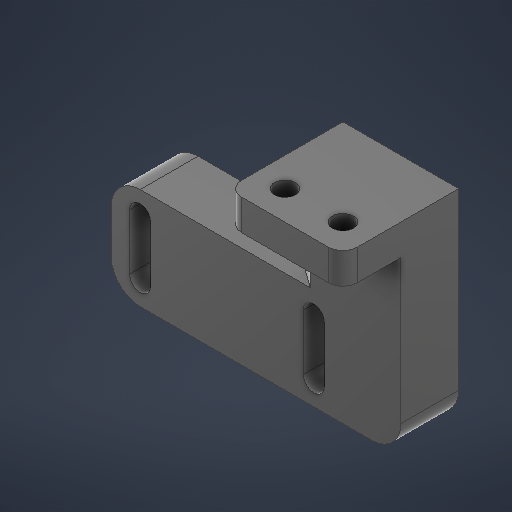
# Autodesk Inventor part: Optical Mount
Saved by Autodesk Inventor 2025 (Build 290162000, 162)
## iProperties
Created: 2024-12-22
Part Number: Optical Mount
Material: Generic
Document SubType Name: Modeling
Designer: Juan
Density: 1 g/cm^3
Appearance: Default
Author: Juan
Autodesk Inventor part; units mm, degrees
ref_plane "YZ Plane" through (0, 0, 0) normal (1, 0, 0) x (0, 1, 0)
ref_plane "XZ Plane" through (0, 0, 0) normal (0, 1, 0) x (-1, 0, 0)
ref_plane "XY Plane" through (0, 0, 0) normal (0, 0, 1) x (1, 0, 0)
sketch "Sketch1" plane through (0, 0, 0) normal (0, 0, 1) x (1, 0, 0)
  line L0 (-19.1352, -8.5102) -> (-19.1352, 8.3898) construction
  line L1 (-16.8111, -6.1861) -> (-16.8111, 6.0657)
  line L2 (-21.4593, 6.0657) -> (-21.4593, -6.1861)
  arc A0 (-21.4593, -6.1861) -> (-16.8111, -6.1861) centre (-19.1352, -6.1861) ccw
  arc A1 (-16.8111, 6.0657) -> (-21.4593, 6.0657) centre (-19.1352, 6.0657) ccw
  line L3 (18.9648, -8.5102) -> (18.9648, 8.3898) construction
  line L4 (21.2889, -6.1861) -> (21.2889, 6.0657)
  line L5 (16.6407, 6.0657) -> (16.6407, -6.1861)
  arc A2 (16.6407, -6.1861) -> (21.2889, -6.1861) centre (18.9648, -6.1861) ccw
  arc A3 (21.2889, 6.0657) -> (16.6407, 6.0657) centre (18.9648, 6.0657) ccw
  line L6 (-19.1352, 8.3898) -> (18.9648, 8.3898)
  line L7 (18.9648, -8.5102) -> (-19.1352, -8.5102)
  line L8 (25.3148, 11.0523) -> (-25.4852, 11.0523)
  line L9 (-25.4852, 11.0523) -> (-25.4852, -11.1727)
  line L10 (-25.4852, -11.1727) -> (25.3148, -11.1727)
  line L11 (25.3148, -11.1727) -> (25.3148, 11.0523)
  line L12 (25.3148, 11.0523) -> (-25.4852, -11.1727) construction
  line L13 (-25.4852, 11.0523) -> (25.3148, -11.1727) construction
  point P0 (0, 0)
  point P1 (-0.0852, -0.0602)
  point P2 (-19.1352, -0.0602)
  point P3 (18.9648, -0.0602)
  dimension "d0" = 4.6482
  dimension "d1" = 4.6482
  dimension "d2" = 50.8
  dimension "d3" = 22.225
  constraints: 32 end point, 12 point on circle, 10 tangent, 5 parallel, 4 centre point, 4 midpoint, 4 point on line, 2 perpendicular, 1 horizontal, 1 other
  measures "d0" diameter of A1
  measures "d1" diameter of A3
  measures "d2" distance of L10.end L9.end
  measures "d3" distance of L9.end L8.end
extrude "Extrusion1" add sketch "Sketch1" along normal blind 12.7 contours L1 A1 L6 A3 L5 A2 L7 A0 | L11 L10 L9 L8
sketch "Sketch2" plane through (-25.4852, 11.0523, 0) normal (0, 1, 0) x (1, 0, 0)
  line L0 (0, 0) -> (50.8, 0) projected
  line L1 (0, 0) -> (12.7, 0)
  line L2 (12.7, 0) -> (12.7, -12.7)
  line L3 (12.7, -12.7) -> (0, -12.7)
  line L4 (0, -12.7) -> (0, 0)
  line L5 (50.8073, 0) -> (38.1073, 0)
  line L6 (38.1073, 0) -> (38.1073, -12.7)
  line L7 (38.1073, -12.7) -> (50.8073, -12.7)
  line L8 (50.8, 0) -> (50.8, -12.7) projected
  line L9 (50.8, 0) -> (50.8, -12.7) projected
  line L10 (50.8, -12.7) -> (50.8, 0)
  line L11 (50.8, 0) -> (38.1073, 0)
  point P0 (25.4852, 0)
  dimension "d7" = 12.7
  dimension "d8" = 12.7
  dimension "d9" = 12.7
  dimension "d10" = 12.7
  constraints: 18 end point, 3 parallel, 3 perpendicular, 3 point on line, 1 collinear
  measures "d7" distance of L2.end L3.end
  measures "d8" distance of L6.end L7.end
  measures "d9" distance of L7.end L5.start
  measures "d10" distance of L3.end L0.start
extrude "Extrusion2" add sketch "Sketch2" along normal blind 22.3933
chamfer "Chamfer1" distance 3.9688 distance2 5.5563 1 edges at (12.6221, 22.2489, 12.7) measured on face at (12.6221, 22.2489, 12.2)
chamfer "Chamfer2" distance 4.7625 distance2 7.9375 1 edges at (-12.7852, 22.2489, 0) measured on face at (-12.7852, 22.2489, 0.5)
sketch "Sketch3" plane through (-25.4852, 33.4456, 0) normal (0, 1, 0) x (1, 0, 0)
  line L0 (0, 0) -> (6.319, 0)
  line L1 (38.1073, 0) -> (4.7625, 0) projected
  line L2 (6.319, -0.6519) -> (0, -0.6519)
  line L3 (0, 0) -> (0, -12.7) projected
  line L4 (0, 0) -> (0, -0.6519)
  line L5 (6.319, 0) -> (6.319, -0.6519)
  point P0 (25.4852, 0)
  constraints: 8 end point, 2 point on line, 1 collinear, 1 parallel, 1 perpendicular
extrude "Extrusion3" cut sketch "Sketch3" against normal up to surface (22.3933 mm away)
fillet "Fillet2" radius 3.175 2 edges at (-19.6363, 22.2489, 0.6519) (-25.4852, 22.2489, 0.6519)
sketch "Sketch4" plane through (0, 0, 12.7) normal (0, 0, 1) x (1, 0, 0)
  line L0 (-12.7852, 11.0523) -> (-18.8822, 11.0523) projected
  line L1 (-12.7852, 11.0523) -> (-12.7852, 26.6987)
  line L2 (-12.7852, 33.4456) -> (-12.7852, 11.0523) projected
  line L3 (-12.7852, 11.0523) -> (25.3148, 11.0523)
  line L4 (25.3148, -11.1727) -> (25.3148, 33.4456) projected
  line L5 (25.3148, 11.0523) -> (25.3148, 26.6987)
  line L6 (12.6221, 33.4456) -> (12.6221, 11.0523) projected
  line L7 (-25.4852, -11.1727) -> (-25.4852, 33.4456) projected
  line L8 (25.3148, 26.6987) -> (12.6221, 26.6987)
  line L9 (12.6221, 26.6987) -> (12.6221, 36.2237)
  line L10 (25.3148, 36.2237) -> (25.3148, 26.6987)
  line L11 (-12.7852, 26.6987) -> (-25.4852, 26.6987)
  line L12 (-25.4852, 26.6987) -> (-25.4852, 36.2237)
  line L13 (-12.7852, 36.2237) -> (-12.7852, 26.6987)
  line L14 (18.1783, 33.4456) -> (12.6221, 33.4456) projected
  line L15 (25.3148, 33.4456) -> (12.6221, 33.4456)
  line L16 (-12.7852, 36.2237) -> (-12.7852, 33.4456)
  line L17 (-25.4852, 33.4456) -> (-12.7852, 33.4456) projected
  line L18 (-12.7852, 33.4456) -> (-25.4852, 33.4456)
  line L19 (-25.4852, 33.4456) -> (-25.4852, 36.2237)
  line L20 (12.6221, 33.4456) -> (12.6221, 26.6987)
  line L21 (25.3148, 26.6987) -> (25.3148, 33.4456)
  line L22 (-12.7852, 26.6987) -> (-12.7852, 33.4456)
  line L23 (-25.4852, 26.6987) -> (-25.4852, 33.4456)
  point P0 (0, 0)
  dimension "d22" = 15.6464
  constraints: 34 end point, 6 perpendicular, 6 point on line, 4 parallel, 3 collinear, 1 horizontal
  measures "d22" distance of L0.start L1.end
extrude "Extrusion4" add sketch "Sketch4" along normal blind 12.7 contours L2 L11 L7 L17 | L6 L14 L15 L4 L8
extrude "Extrusion5" add sketch "Sketch4" against normal blind 4.2333 contours L6 L14 L15 L4 L8
sketch "Sketch5" plane through (-25.4852, 33.4456, 0) normal (0, 1, 0) x (1, 0, 0)
  line L0 (50.8, -25.4) -> (38.1073, -25.4) projected
  line L1 (12.7, -25.4) -> (0, -25.4) projected
  line L2 (44.4537, -25.4) -> (44.4537, -19.05)
  line L3 (6.35, -25.4) -> (6.35, -19.05)
  circle A0 centre (6.35, -19.05) radius 2.3241
  circle A1 centre (44.4537, -19.05) radius 2.3241
  point P0 (25.4852, 0)
  dimension "d27" = 6.35
  dimension "d28" = 6.35
  dimension "d29" = 4.6482
  dimension "d30" = 4.6482
  constraints: 4 end point, 2 centre point, 2 coincident, 2 midpoint, 2 vertical
  measures "d27" distance of L2.start L2.end
  measures "d28" distance of L3.start L3.end
  measures "d29" diameter of A0
  measures "d30" diameter of A1
extrude "Extrusion6" cut sketch "Sketch5" against normal through all
sketch "Sketch6" plane through (-12.7852, 11.0523, 12.7) normal (1, 0, 0) x (0, 0, -1)
  line L0 (-12.7, 15.6464) -> (-12.7, 22.3933) projected
  line L1 (0, 15.6464) -> (-12.7, 15.6464) projected
  line L2 (-12.7, 15.6464) -> (-12.7, 22.3933)
  line L3 (-12.7, 22.3933) -> (0, 22.3933)
  line L4 (0, 22.3933) -> (0, 15.6464)
  line L5 (0, 15.6464) -> (-12.7, 15.6464)
  point P0 (12.7, -11.0523)
  constraints: 8 end point, 3 equal length, 1 perpendicular
extrude "Extrusion7" [suppressed]
sketch "Sketch7" plane through (18.1783, 26.6987, 12.7) normal (0, -1, 0) x (1, 0, 0)
  circle A0 centre (-37.3136, 6.35) radius 2.3241 projected
  circle A1 centre (0.7901, 6.35) radius 2.3241 projected
  line L0 (-37.3136, 6.35) -> (-24.6136, 6.35)
  line L1 (-24.6136, 6.35) -> (-11.9136, 6.35)
  line L2 (-26.798, 4.1656) -> (-22.4292, 4.1656)
  line L3 (-22.4292, 4.1656) -> (-22.4292, 8.5344)
  line L4 (-22.4292, 8.5344) -> (-26.798, 8.5344)
  line L5 (-26.798, 8.5344) -> (-26.798, 4.1656)
  line L6 (-26.798, 4.1656) -> (-22.4292, 8.5344) construction
  line L7 (-22.4292, 4.1656) -> (-26.798, 8.5344) construction
  line L8 (-9.7292, 8.5344) -> (-14.098, 8.5344)
  line L9 (-9.7292, 4.1656) -> (-9.7292, 8.5344)
  line L10 (-14.098, 4.1656) -> (-9.7292, 4.1656)
  line L11 (-14.098, 8.5344) -> (-14.098, 4.1656)
  point P0 (-18.1783, -12.7)
  dimension "d35" = 12.7
  dimension "d36" = 12.7
  dimension "d37" = 4.3688
  dimension "d38" = 4.3688
  dimension "d41" = 12.7
  constraints: 24 end point, 3 horizontal, 2 midpoint, 2 parallel, 1 perpendicular, 1 point on line, 8 other
  measures "d35" distance of L0.start L0.end
  measures "d36" distance of L0.end L1.end
  measures "d37" distance of L4.end L3.end
  measures "d38" distance of L3.end L2.end
  measures "d41" distance of L3.end L8.start
extrude "Extrusion8" [suppressed]
fillet "Fillet3" [suppressed]
sketch "Sketch8" plane through (-25.4852, 11.0523, 0) normal (0, 1, 0) x (1, 0, 0)
  line L0 (38.1073, 0) -> (0, 0) projected
  line L1 (0, 0) -> (14.6548, 0)
  line L2 (14.6548, 0) -> (14.6548, -26.951)
  line L3 (14.6548, -26.951) -> (0, -26.951)
  line L4 (0, -26.951) -> (0, 0)
  point P0 (25.4852, 0)
  point P1 (14.6548, 0)
  constraints: 8 end point, 2 parallel, 1 horizontal, 1 perpendicular
extrude "Extrusion9" cut sketch "Sketch8" along normal blind 25.4
sketch "Sketch9" plane through (25.3148, -11.1727, 12.7) normal (1, 0, 0) x (0, 0, -1)
  line L0 (0, 0) -> (0, 37.8714) projected
  line L1 (12.7, 0) -> (0, 0) projected
  line L2 (12.7, 0) -> (12.7, 44.6183) projected
  line L3 (12.7, 44.6183) -> (-12.7, 44.6183) projected
  line L4 (-12.7, 37.8714) -> (-12.7, 44.6183) projected
  line L5 (0, 37.8714) -> (-12.7, 37.8714) projected
  point P0 (12.7, 11.1727)
extrude "Extrusion10" add sketch "Sketch9" along normal blind 12.7
sketch "Sketch10" plane through (-25.4852, 33.4456, 0) normal (0, 1, 0) x (1, 0, 0)
  circle A0 centre (44.4537, -19.05) radius 2.3241 projected
  line L0 (44.4537, -19.05) -> (57.1537, -19.05)
  circle A1 centre (57.1537, -19.05) radius 2.3241
  point P0 (25.4852, 0)
  dimension "d58" = 12.7
  dimension "d59" = 4.6482
  constraints: 2 end point, 1 centre point, 1 coincident, 1 horizontal
  measures "d58" distance of L0.start L0.end
  measures "d59" diameter of A1
extrude "Extrusion11" cut sketch "Sketch10" against normal blind 12.7 contours A1
fillet "Fillet9" radius 3.175 2 edges at (12.6221, 30.0721, 25.4) (38.0148, 30.0721, 25.4)
fillet "Fillet10" radius 6.35 3 edges at (-25.4852, 11.0523, 6.35) (-25.4852, -11.1727, 6.35) (38.0148, -11.1727, 6.35)
body "Solid1"
